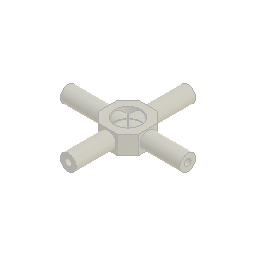
Quad Arm Adaptor (Autodesk Fusion 360 design; units mm, degrees)
Autodesk Fusion 360 part; units mm, degrees
note: some values were not read from the file. Chosen so that the rebuilt part matches the saved one: which face or edge a step refers to.
sketch "Base" plane through (0, 0, 0) normal (0, 0, 1) x (1, 0, 0)
  line L0 (-7, -15) -> (7, -15)
  line L1 (7, -15) -> (15, -7)
  line L2 (15, -7) -> (15, 7)
  line L3 (15, 7) -> (7, 15)
  line L4 (7, 15) -> (-7, 15)
  line L5 (-7, 15) -> (-15, 7)
  line L6 (-15, 7) -> (-15, -7)
  line L7 (-15, -7) -> (-7, -15)
  circle A0 centre (0, 0) radius 10
  point P0 (0, 15)
  point P1 (-15, 0)
  point P2 (0, -15)
  point P3 (15, 0)
  point P4 (-11, 11)
  point P5 (-11, -11)
  point P6 (11, -11)
  dimension "d12" = 14
  dimension "d13" = 14
  dimension "d14" = 14
  dimension "d15" = 14
  dimension "d16" = 30
  dimension "d17" = 15
  dimension "d18" = 30
  dimension "d19" = 15
  dimension "d82" = 20
  constraint horizontal L0
  constraint vertical L2
  constraint perpendicular L2 L4
  constraint parallel L2 L6
  constraint midpoint L4 P0
  constraint midpoint L6 P1
  constraint midpoint L0 P2
  constraint midpoint L2 P3
  constraint coincident A0.centre origin
  measures "d12" distance of L0.start L0.end
  measures "d13" distance of L1.end L2.end
  measures "d14" distance of L3.end L4.end
  measures "d15" distance of L5.end L6.end
  measures "d16" distance of L2 L6
  measures "d17" distance of L6 P2
  measures "d18" distance of L0 L4
  measures "d19" distance of L0 P3
  measures "d82" diameter of A0
extrude "Extrude1" add sketch "Base" along normal blind 14
sketch "Arm Adaptor 1" plane through (0, 0, 0) normal (0, 1, 0) x (1, 0, 0)
  line L0 (-7, -14) -> (7, -14)
  line L1 (7, -14) -> (7, 0)
  line L2 (7, 0) -> (-7, 0)
  line L3 (-7, 0) -> (-7, -14)
  circle A0 centre (0, -7) radius 6
  circle A1 centre (0, -7) radius 2.5
  dimension "d67" = 12
  dimension "d68" = 5
  constraint horizontal L0
  constraint vertical L1
  constraint horizontal L2
  constraint vertical L3
  constraint concentric A0 A1
  measures "d67" diameter of A0
  measures "d68" diameter of A1
extrude "Extrude5" add sketch "Arm Adaptor 1" along normal blind -30 and the other way blind -15 from surface at -15 contours A0
extrude "Extrude6" add sketch "Arm Adaptor 1" along normal blind 30 and the other way blind 15 from surface at 15 contours A0
sketch "Arm Adaptor 2" plane through (0, 0, 0) normal (1, 0, 0) x (0, 1, 0)
  line L0 (-7, 14) -> (7, 14)
  line L1 (7, 14) -> (7, 0)
  line L2 (7, 0) -> (-7, 0)
  line L3 (-7, 0) -> (-7, 14)
  circle A0 centre (0, 7) radius 6
  circle A1 centre (0, 7) radius 2.5
  dimension "d69" = 12
  dimension "d70" = 5
  constraint horizontal L0
  constraint vertical L1
  constraint horizontal L2
  constraint vertical L3
  constraint concentric A0 A1
  measures "d69" diameter of A0
  measures "d70" diameter of A1
extrude "Extrude8" add sketch "Arm Adaptor 2" along normal blind 30 and the other way blind 15 from surface at 15 contours A0
extrude "Extrude9" add sketch "Arm Adaptor 2" along normal blind -30 and the other way blind -15 from surface at -15 contours A0
extrude "Extrude12" cut sketch "Arm Adaptor 1" along normal through all and the other way through all contours A1
extrude "Extrude13" cut sketch "Arm Adaptor 2" along normal through all and the other way through all contours A1
fillet "Fillet3" radius 1 7 edges at (-4.2426, 4.2426, 11.2426) (-6, -6, 7) (-4.2426, 4.2426, 2.7574) (4.2426, 4.2426, 11.2426) (4.2426, 4.2426, 2.7574) (4.2426, -4.2426, 11.2426) (4.2426, -4.2426, 2.7574)
equation "d17 = d16 / 2"
equation "d18 = d16"
equation "d19 = d18 / 2"
named bodies: "Quad Arm Adaptor"
